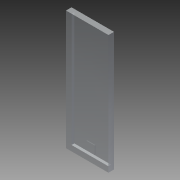
# Autodesk Inventor part: YagiCan
Saved by Autodesk Inventor 2014 (Build 180170000, 170)
## iProperties
Created: 2015-04-15
Part Number: YagiCan
Material: Generic
Document SubType Name: Modeling
Designer: Owner
Density: 1 g/cm^3
Appearance: Clear
Author: Owner
Autodesk Inventor part; units mm, degrees
ref_plane "YZ Plane" through (0, 0, 0) normal (1, 0, 0) x (0, 1, 0)
ref_plane "XZ Plane" through (0, 0, 0) normal (0, 1, 0) x (-1, 0, 0)
ref_plane "XY Plane" through (0, 0, 0) normal (0, 0, 1) x (1, 0, 0)
sketch "Sketch1" plane through (0, 0, 0) normal (0, 0, 1) x (1, 0, 0)
  line L0 (-13.3613, 31.5734) -> (9.3717, 31.5734)
  line L1 (9.3717, 31.5734) -> (9.3717, -35.1016)
  line L2 (9.3717, -35.1016) -> (-13.3613, -35.1016)
  line L3 (-13.3613, -35.1016) -> (-13.3613, 31.5734)
  line L4 (10.1591, 32.3608) -> (-14.1487, 32.3608)
  line L5 (-14.1487, 32.3608) -> (-14.1487, -35.889)
  line L6 (-14.1487, -35.889) -> (10.1591, -35.889)
  line L7 (10.1591, -35.889) -> (10.1591, 32.3608)
  line L8 (8.5843, 30.786) -> (-12.5739, 30.786)
  line L9 (-12.5739, 30.786) -> (-12.5739, -34.3142)
  line L10 (-12.5739, -34.3142) -> (8.5843, -34.3142)
  line L11 (8.5843, -34.3142) -> (8.5843, 30.786)
  point P0 (0, 0)
  dimension "d0" = 22.733
  dimension "d1" = 66.675
  dimension "d2" = 0.7874
  dimension "d3" = 0.7874
  constraints: 24 end point, 6 parallel, 3 perpendicular, 1 horizontal, 6 other
  measures "d0" distance of L0.start L0.end
  measures "d1" distance of L0.end L1.end
  measures "d2" distance between parallel lines of L0 L4
  measures "d3" distance between parallel lines of L8 L0
extrude "Extrusion1" add sketch "Sketch1" along normal blind 1.5875 contours L0 L1 L2 L3 | L7 L6 L5 L4
sketch "Sketch3" plane through (0, 0, 1.5875) normal (0, 0, 1) x (1, 0, 0)
  line L0 (-14.1487, 32.3608) -> (10.1591, 32.3608)
  line L1 (10.1591, 32.3608) -> (10.1591, -35.889)
  line L2 (10.1591, -35.889) -> (-14.1487, -35.889)
  line L3 (-14.1487, -35.889) -> (-14.1487, 32.3608)
  point P0 (0, 0)
  constraints: 8 end point, 2 parallel, 1 horizontal, 1 perpendicular
extrude "Extrusion2" add sketch "Sketch3" along normal blind 1.5875
sketch "Sketch4" plane through (0, 0, 1.5875) normal (0, 0, -1) x (-1, 0, 0)
  line L0 (1.1699, -25.422) -> (5.9324, -25.422)
  line L1 (5.9324, -25.422) -> (5.9324, -30.1845)
  line L2 (5.9324, -30.1845) -> (1.1699, -30.1845)
  line L3 (1.1699, -30.1845) -> (1.1699, -25.422)
  point P0 (0, 0)
  dimension "d10" = 4.7625
  dimension "d11" = 4.7625
  constraints: 8 end point, 2 parallel, 1 horizontal, 1 perpendicular
  measures "d10" distance of L0.end L1.end
  measures "d11" distance of L0.start L0.end
extrude "Extrusion3" add sketch "Sketch4" along normal blind 0.508
body "Solid1"
